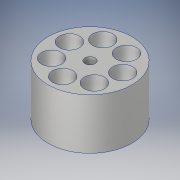
# Autodesk Inventor part: Flywheel
Saved by Autodesk Inventor 2019.4 (Build 234330000, 330)
## iProperties
Created: 2020-01-06
Part Number: Flywheel
Material: Aluminum 6061
Document SubType Name: Modeling
Designer: admin
Density: 2.7 g/cm^3
Appearance: Aluminum - Flat
Mass: 711.93 g
Surface Area: 250.848 cm^2
Volume: 263.678 cm^3
Author: admin
Autodesk Inventor part; units mm, degrees
ref_plane "YZ Plane" through (0, 0, 0) normal (1, 0, 0) x (0, 1, 0)
ref_plane "XZ Plane" through (0, 0, 0) normal (0, 1, 0) x (-1, 0, 0)
ref_plane "XY Plane" through (0, 0, 0) normal (0, 0, 1) x (1, 0, 0)
sketch "Sketch1" plane through (0, 0, 0) normal (0, 1, 0) x (-1, 0, 0)
  circle A0 centre (0, 0) radius 41.275
  circle A1 centre (0, 0) radius 5
  dimension "d0" = 10
  dimension "d1" = 82.55
  constraints: 2 centre point, 2 coincident
  measures "d0" diameter of A1
  measures "d1" diameter of A0
extrude "Extrusion1" add sketch "Sketch1" along normal blind 50
sketch "Sketch2" plane through (0, 50, 0) normal (0, 1, 0) x (1, 0, 0)
  circle A0 centre (0, -27) radius 10
  line L0 (0, -27) -> (0, 0) construction
  circle A1 centre (21.1095, -16.8342) radius 10
  circle A2 centre (26.3231, 6.0081) radius 10
  circle A3 centre (11.7149, 24.3262) radius 10
  circle A4 centre (-11.7149, 24.3262) radius 10
  circle A5 centre (-26.3231, 6.0081) radius 10
  circle A6 centre (-21.1095, -16.8342) radius 10
  dimension "d4" = 20
  dimension "d5" = 27
  dimension "d8" = 360
  constraints: 7 centre point, 2 end point, 1 vertical, 15 other
  measures "d4" diameter of A0
  measures "d5" distance of L0.start L0.end
extrude "Extrusion2" cut sketch "Sketch2" against normal through all
body "Solid1"
